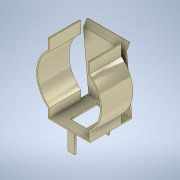
# Autodesk Inventor part: AA-Cell-Holder
Saved by Autodesk Inventor 2022 (Build 260153000, 153)
## iProperties
Created: 2024-06-20
Part Number: AA-Cell-Holder
Material: 一般
Document SubType Name: Modeling
Designer: yamashita1
Density: 1 g/cm^3
Appearance: ニッケル
Author: yamashita1
Autodesk Inventor part; units mm, degrees
sketch "スケッチ1" plane through (0, 0, 0) normal (0, 1, 0) x (-1, 0, 0)
  line L0 (4.5, -0.3) -> (-4.5, -0.3)
  line L1 (-4.5, -0.3) -> (-4.5, 0)
  line L2 (-4.5, 0) -> (4.5, 0)
  line L3 (4.5, 0) -> (4.5, -0.3)
  line L4 (9.7545, -2) -> (-9.7545, -2) construction
  line L5 (0, -25.3634) -> (0, 2.8638) construction
  circle A0 centre (0, -7.3619) radius 7
  circle A1 centre (0, -7.3619) radius 6.7
  line L6 (4.5, -0.3) -> (4.5, -2)
  line L7 (4.2, -0.3) -> (4.2, -2.1417)
  line L8 (-4.5, -0.3) -> (-4.5, -2)
  line L9 (-4.2, -0.3) -> (-4.2, -2.1417)
  line L10 (9.7545, -15) -> (-9.7545, -15) construction
  line L11 (4.5, -12.7238) -> (4.5, -15)
  line L12 (4.5, -15) -> (4.2, -15)
  line L13 (4.2, -12.5821) -> (4.2, -15)
  line L14 (-4.5, -12.7238) -> (-4.5, -15)
  line L15 (-4.5, -15) -> (-4.2, -15)
  line L16 (-4.2, -15) -> (-4.2, -12.5821)
  point P0 (0, 0)
  point P1 (0, 0)
  point P2 (0, -2)
  point P3 (0, -15)
  dimension "d0" = 9
  dimension "THIN" = 0.3
  dimension "d2" = 2
  dimension "d3" = 14
  dimension "d5" = 0.3
  dimension "d6" = 0.3
  dimension "d7" = 0.3
  dimension "d8" = 15
  constraints: 34 end point, 11 point on line, 8 point on circle, 6 perpendicular, 5 parallel, 4 collinear, 3 horizontal, 3 midpoint, 2 centre point, 2 coincident, 1 vertical
  measures "d0" distance of L1.end L2.end
  measures "THIN" distance of L0.end L1.end
  measures "d2" distance from line of point (0, 0) L4
  measures "d3" diameter of A0
  measures "d5" radial gap between concentric circles of A0 A1
  measures "d6" distance between parallel lines of L7 L6
  measures "d7" distance between parallel lines of L8 L9
  measures "d8" distance from line of point (0, 0) L10
extrude "押し出し1" add sketch "スケッチ1" along normal blind 6.7 contours L6 A0 L7 L0 | L0 L1 L2 L3 | A0 L13 A1 L7 | L9 A0 L8 L0 | L9 A1 L16 A0 | L11 L12 L13 A0 | A0 L16 L15 L14
sketch "スケッチ2" plane through (0, 0, 0) normal (0, -1, 0) x (1, 0, 0)
  line L0 (4.5, 0) -> (4.5, -2) projected
  line L1 (-4.5, -2) -> (-4.5, 0) projected
  line L2 (4.5, 0) -> (-4.5, 0)
  line L3 (-4.5, 0) -> (-4.5, -0.3)
  line L4 (-4.5, -0.3) -> (4.5, -0.3)
  line L5 (4.5, -0.3) -> (4.5, 0)
  line L6 (4.2, -0.3) -> (-4.2, -0.3) projected
  point P0 (0, 0)
  point P1 (4.5, -0.3)
  constraints: 8 end point, 2 parallel, 1 collinear, 1 horizontal, 1 perpendicular, 1 point on line
extrude "押し出し2" add sketch "スケッチ2" along normal blind 2.3
ref_plane "作業平面1" through (-4.5, -2.3, -0.3) normal (0, 0.9962, 0.0872) x (1, 0, 0)
sketch "スケッチ3" plane through (-4.5, -2.3, -0.3) normal (0, 0.9962, 0.0872) x (1, 0, 0)
  line L0 (0, 0) -> (9, 0) projected
  line L1 (9, 0) -> (0, 0)
  line L2 (0, 0) -> (0, 13)
  line L3 (0, 13) -> (9, 13)
  line L4 (9, 13) -> (9, 0)
  point P0 (4.5, -0.0984)
  dimension "d14" = 13
  constraints: 8 end point, 2 parallel, 1 horizontal, 1 perpendicular
  measures "d14" distance of L0.start L2.end
extrude "押し出し3" add sketch "スケッチ3" along normal blind 0.3
ref_plane "作業平面2" through (4.5, -0.8681, -13.2244) normal (0, -0.8387, 0.5446) x (-1, 0, 0)
sketch "スケッチ4" plane through (4.5, -0.8681, -13.2244) normal (0, -0.8387, 0.5446) x (-1, 0, 0)
  line L0 (9, 0) -> (9, -10.2235) projected
  line L1 (9, 0) -> (0, 0)
  line L2 (0, 0) -> (0, 1.5)
  line L3 (0, 1.5) -> (9, 1.5)
  line L4 (9, 1.5) -> (9, 0)
  point P0 (4.5, -11.5637)
  dimension "d18" = 1.5
  constraints: 8 end point, 2 parallel, 1 coincident, 1 horizontal, 1 perpendicular
  measures "d18" distance of L1.end L2.end
extrude "押し出し4" add sketch "スケッチ4" along normal blind 0.3
sketch "スケッチ5" plane through (4.2, 6.7, -0.3) normal (0, 0, -1) x (-1, 0, 0)
  line L0 (5.95, -2) -> (2.45, -2)
  line L1 (2.45, -2) -> (2.45, -7.7)
  line L2 (2.45, -7.7) -> (5.95, -7.7)
  line L3 (5.95, -7.7) -> (5.95, -2)
  line L4 (0, 0) -> (8.4, 0) projected
  point P0 (4.2, -6.7)
  point P1 (4.2, -7.7)
  dimension "d21" = 2
  dimension "d22" = 3.5
  dimension "d23" = 5.7
  constraints: 8 end point, 2 parallel, 1 horizontal, 1 midpoint, 1 perpendicular, 1 vertical alignment
  measures "d21" distance between parallel lines of L4 L0
  measures "d22" distance of L0.start L0.end
  measures "d23" distance of L0.end L1.end
extrude "押し出し5" cut sketch "スケッチ5" against normal through all
sketch "スケッチ7" plane through (-1.75, -1, -0.3) normal (0, 1, 0) x (1, 0, 0)
  line L0 (3.5, -0.3) -> (0, -0.3) projected
  line L1 (1, -0.3) -> (2.5, -0.3)
  line L2 (2.5, -0.3) -> (2.5, -4.7)
  line L3 (2.5, -4.7) -> (1, -4.7)
  line L4 (1, -4.7) -> (1, -0.3)
  point P0 (1.75, -0.3)
  point P1 (1.75, -0.3)
  dimension "d30" = 1.5
  dimension "d31" = 4.4
  constraints: 8 end point, 2 midpoint, 2 parallel, 1 horizontal, 1 perpendicular, 1 point on line
  measures "d30" distance of L2.end L3.end
  measures "d31" distance of L1.end L2.end
extrude "押し出し7" add sketch "スケッチ7" against normal blind 0.3
ref_plane "作業平面3" through (0, 6.2, 0) normal (0, 1, 0) x (1, 0, 0)
sketch "スケッチ8" plane through (0, 6.2, 0) normal (0, 1, 0) x (1, 0, 0)
  line L0 (4.5, 0) -> (-4.5, 0) projected
  line L1 (-0.75, 0) -> (0.75, 0)
  line L2 (0.75, 0) -> (0.75, -4.4)
  line L3 (0.75, -4.4) -> (-0.75, -4.4)
  line L4 (-0.75, -4.4) -> (-0.75, 0)
  line L5 (-4.5, 0) -> (4.5, 0) projected
  point P0 (0, 0)
  point P1 (0, -4.4)
  point P2 (0, 0)
  dimension "d35" = 1.5
  dimension "d36" = 4.4
  constraints: 8 end point, 2 midpoint, 2 parallel, 1 horizontal, 1 perpendicular, 1 point on line, 1 vertical alignment
  measures "d35" distance of L2.end L3.end
  measures "d36" distance of L1.end L2.end
extrude "押し出し8" add sketch "スケッチ8" against normal blind 0.3
equation "\"d5\" = THIN"
equation "\"d6\" = THIN"
equation "\"d7\" = THIN"
equation "\"d15\" = THIN"
equation "\"d19\" = THIN"
equation "\"d32\" = THIN"
equation "\"d37\" = THIN"
